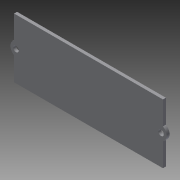
# Autodesk Inventor part: power channel cap
Saved by Autodesk Inventor 2014 SP1 (Build 180222100, 222)
## iProperties
Created: 2017-08-02
Part Number: power channel cap
Material: Generic
Document SubType Name: Modeling
Designer: kteo17
Density: 1 g/cm^3
Appearance: Default
Author: kteo17
Autodesk Inventor part; units mm, degrees
ref_plane "YZ Plane" through (0, 0, 0) normal (1, 0, 0) x (0, 1, 0)
ref_plane "XZ Plane" through (0, 0, 0) normal (0, 1, 0) x (-1, 0, 0)
ref_plane "XY Plane" through (0, 0, 0) normal (0, 0, 1) x (1, 0, 0)
sketch "Sketch1" plane through (0, 0, 0) normal (0, 0, 1) x (1, 0, 0)
  line L0 (0, 0) -> (63.5, 0)
  line L1 (63.5, 25.4) -> (0, 25.4)
  arc A0 (0, 15.4496) -> (0, 9.9504) centre (1.5875, 12.7) ccw
  arc A1 (63.5, 9.9504) -> (63.5, 15.4496) centre (61.9125, 12.7) ccw
  circle A2 centre (0.7937, 12.7) radius 1.1938
  circle A3 centre (62.7062, 12.7) radius 1.1938
  line L2 (0, 25.4) -> (0, 15.4496)
  line L3 (0, 9.9504) -> (0, 0)
  line L4 (63.5, 0) -> (63.5, 9.9504)
  line L5 (63.5, 15.4496) -> (63.5, 25.4)
  dimension "d0" = 63.5
  dimension "d1" = 25.4
  dimension "d4" = 2.3876
  dimension "d5" = 2.3876
  constraints: 12 end point, 5 parallel, 4 centre point, 4 point on circle, 2 perpendicular, 1 horizontal
  measures "d0" distance of L1.end L1.start
  measures "d1" distance of L1.start L0.end
  measures "d4" diameter of A2
  measures "d5" diameter of A3
extrude "Extrusion1" add sketch "Sketch1" along normal blind 1.27
body "Solid1"
